Autodesk Inventor part; units mm, degrees
(part 2 of 2)
  spline S15 degree 2 poles (-9.398, 4.6838) (-9.0358, 4.6838) (-8.2948, 4.8649) (-7.9572, 5.0049) knots 0 0 0 1 2 2 2
  spline S16 degree 2 poles (-7.9572, 5.0049) (-7.669, 5.1202) (-7.1338, 5.4495) (-6.9692, 5.5648) knots 0 0 0 1 2 2 2
  line L105 (-6.9692, 5.5648) -> (-6.8951, 5.5648)
  line L106 (-6.8951, 5.5648) -> (-6.8951, 4.1157)
  spline S17 degree 2 poles (-6.8951, 4.1157) (-7.315, 3.9099) (-8.8217, 3.5064) (-9.4968, 3.5064) knots 0 0 0 1 2 2 2
  spline S18 degree 2 poles (-9.4968, 3.5064) (-10.9212, 3.5064) (-12.5267, 5.0131) (-12.5267, 6.2975) knots 0 0 0 1 2 2 2
  spline S19 degree 2 poles (-12.5267, 6.2975) (-12.5267, 6.8986) (-12.2468, 7.9031) (-11.9998, 8.3312) knots 0 0 0 1 2 2 2
  spline S20 degree 2 poles (-11.9998, 8.3312) (-11.7528, 8.7758) (-11.0365, 9.6485) (-10.6413, 10.0684) knots 0 0 0 1 2 2 2
  spline S21 degree 2 poles (-10.6413, 10.0684) (-9.9991, 10.7683) (-8.4265, 12.2668) (-7.9572, 12.7031) knots 0 0 0 1 2 2 2
  line L107 (-7.9572, 12.7031) -> (-12.9466, 12.7031)
  line L108 (-12.9466, 12.7031) -> (-12.9466, 13.8805)
  line L109 (-50.5534, 75.3641) -> (-56.819, 75.3641)
  line L110 (-56.819, 75.3641) -> (-56.819, 76.8049)
  spline S22 degree 2 poles (-56.819, 76.8049) (-56.1439, 77.4389) (-54.9418, 78.6163) (-54.3654, 79.2502) knots 0 0 0 1 2 2 2
  spline S23 degree 2 poles (-54.3654, 79.2502) (-53.2045, 80.5264) (-52.3565, 82.0578) (-52.3565, 82.8729) knots 0 0 0 1 2 2 2
  spline S24 degree 2 poles (-52.3565, 82.8729) (-52.3565, 83.3011) (-52.62, 83.9433) (-52.8587, 84.1491) knots 0 0 0 1 2 2 2
  spline S25 degree 2 poles (-52.8587, 84.1491) (-53.0975, 84.3549) (-53.7232, 84.5608) (-54.102, 84.5608) knots 0 0 0 1 2 2 2
  spline S26 degree 2 poles (-54.102, 84.5608) (-54.4642, 84.5608) (-55.2052, 84.3796) (-55.5428, 84.2397) knots 0 0 0 1 2 2 2
  spline S27 degree 2 poles (-55.5428, 84.2397) (-55.831, 84.1244) (-56.3662, 83.7951) (-56.5308, 83.6798) knots 0 0 0 1 2 2 2
  line L111 (-56.5308, 83.6798) -> (-56.6049, 83.6798)
  line L112 (-56.6049, 83.6798) -> (-56.6049, 85.1289)
  spline S28 degree 2 poles (-56.6049, 85.1289) (-56.185, 85.3347) (-54.6783, 85.7381) (-54.0032, 85.7381) knots 0 0 0 1 2 2 2
  spline S29 degree 2 poles (-54.0032, 85.7381) (-52.5788, 85.7381) (-50.9733, 84.2314) (-50.9733, 82.947) knots 0 0 0 1 2 2 2
  spline S30 degree 2 poles (-50.9733, 82.947) (-50.9733, 82.346) (-51.2532, 81.3415) (-51.5002, 80.9134) knots 0 0 0 1 2 2 2
  spline S31 degree 2 poles (-51.5002, 80.9134) (-51.7472, 80.4688) (-52.4635, 79.596) (-52.8587, 79.1761) knots 0 0 0 1 2 2 2
  spline S32 degree 2 poles (-52.8587, 79.1761) (-53.5009, 78.4763) (-55.0735, 76.9778) (-55.5428, 76.5415) knots 0 0 0 1 2 2 2
  line L113 (-55.5428, 76.5415) -> (-50.5534, 76.5415)
  line L114 (-50.5534, 76.5415) -> (-50.5534, 75.3641)
  line L115 (-12.9466, 13.8805) -> (-6.681, 13.8805)
  line L116 (-6.681, 13.8805) -> (-6.681, 12.4397)
  spline S33 degree 2 poles (-6.681, 12.4397) (-7.3561, 11.8057) (-8.5582, 10.6283) (-9.1346, 9.9943) knots 0 0 0 1 2 2 2
  spline S34 degree 2 poles (-9.1346, 9.9943) (-10.2955, 8.7182) (-11.1435, 7.1868) (-11.1435, 6.3716) knots 0 0 0 1 2 2 2
  spline S35 degree 2 poles (-11.1435, 6.3716) (-11.1435, 5.9435) (-10.88, 5.3013) (-10.6413, 5.0955) knots 0 0 0 1 2 2 2
  spline S36 degree 2 poles (-10.6413, 5.0955) (-10.4025, 4.8896) (-9.7768, 4.6838) (-9.398, 4.6838) knots 0 0 0 1 2 2 2
  spline S37 degree 2 poles (-9.398, 4.6838) (-9.0358, 4.6838) (-8.2948, 4.8649) (-7.9572, 5.0049) knots 0 0 0 1 2 2 2
  spline S38 degree 2 poles (-7.9572, 5.0049) (-7.669, 5.1202) (-7.1338, 5.4495) (-6.9692, 5.5648) knots 0 0 0 1 2 2 2
  line L117 (-6.9692, 5.5648) -> (-6.8951, 5.5648)
  line L118 (-6.8951, 5.5648) -> (-6.8951, 4.1157)
  spline S39 degree 2 poles (-6.8951, 4.1157) (-7.315, 3.9099) (-8.8217, 3.5064) (-9.4968, 3.5064) knots 0 0 0 1 2 2 2
  spline S40 degree 2 poles (-9.4968, 3.5064) (-10.9212, 3.5064) (-12.5267, 5.0131) (-12.5267, 6.2975) knots 0 0 0 1 2 2 2
  spline S41 degree 2 poles (-12.5267, 6.2975) (-12.5267, 6.8986) (-12.2468, 7.9031) (-11.9998, 8.3312) knots 0 0 0 1 2 2 2
  spline S42 degree 2 poles (-11.9998, 8.3312) (-11.7528, 8.7758) (-11.0365, 9.6485) (-10.6413, 10.0684) knots 0 0 0 1 2 2 2
  spline S43 degree 2 poles (-10.6413, 10.0684) (-9.9991, 10.7683) (-8.4265, 12.2668) (-7.9572, 12.7031) knots 0 0 0 1 2 2 2
  line L119 (-7.9572, 12.7031) -> (-12.9466, 12.7031)
  line L120 (-12.9466, 12.7031) -> (-12.9466, 13.8805)
  point P0 (-31.75, 68.8958)
  point P1 (-31.75, 20.0009)
  point P2 (-53.7479, 68.8958)
  point P3 (-9.7521, 20.0042)
  point P4 (-13.4723, 102.9238)
  point P5 (-31.75, 68.8958)
  point P6 (-31.75, 20.0009)
  point P7 (-53.7479, 68.8958)
  point P8 (-9.7521, 20.0042)
  dimension "d103" = 8.4153
  dimension "d105" = 0.508
  dimension "d106" = 0.508
  constraints: 220 point on circle, 170 end point, 120 centre point, 20 perpendicular, 20 tangent, 8 vertical, 4 horizontal, 2 midpoint, 1 parallel, 4 other
  measures "d103" distance of L12.end L14.start
  measures "d105" distance between parallel lines of L15 L7
  measures "d106" distance between parallel lines of L16 L11
extrude "Extrusion20" add sketch "Sketch17" along normal blind 0.4 contours L40 A34 A33 A32 L39 L38 L37 L36 A31 A30 A29 A28 A27 L35 A26 L34 A25 A24 L33 | L56 A58 A57 A56 L55 L54 L53 L52 A55 A54 A53 A52 A51 L51 A50 L50 A49 A48 L49 | L72 A82 A81 A80 L71 L70 L69 L68 A79 A78 A77 A76 A75 L67 A74 L66 A73 A72 L65 | L92 A113 A112 L95 L96 A116 A117 A115 L93 L89 L91 L94 A111 A110 A108 A114 A109 L90 A107 | L97 L98 S0 S1 S2 S3 S4 S5 L99 L100 S6 S7 S8 S9 S10 L101 L102 | L103 L104 S11 S12 S13 S14 S15 S16 L105 L106 S17 S18 S19 S20 S21 L107 L108 bodies 1
sketch "Sketch18" plane through (0, 0, -0.2) normal (0, 0, -1) x (-1, 0, 0)
  line L0 (0, 0) -> (-63.5, 0)
  line L1 (-63.5, 0) -> (-63.5, 88.9)
  line L2 (-63.5, 88.9) -> (0, 88.9)
  line L3 (0, 88.9) -> (0, 0)
  constraints: 8 end point, 2 parallel, 1 horizontal, 1 perpendicular
extrude "Extrusion21" add sketch "Sketch18" along normal blind 0.4 bodies 3
fillet "Fillet2" radius 3.175 8 edges at (63.5, 0, 0.2) (63.5, 88.9, 0.2) (0, 0, 0.2) (0, 88.9, 0.2) (63.5, 0, -0.3) (63.5, 88.9, -0.3) (0, 0, -0.3) (0, 88.9, -0.3)
extrude "Extrusion22" cut sketch "Sketch17" along normal blind 0.4 contours L40 A34 A33 A32 L39 L38 L37 L36 A31 A30 A29 A28 A27 L35 A26 L34 A25 A24 L33 | L44 A41 A40 L47 L48 A44 A45 A43 L45 L41 L43 L46 A39 A38 A36 A42 A37 L42 A35 | L56 A58 A57 A56 L55 L54 L53 L52 A55 A54 A53 A52 A51 L51 A50 L50 A49 A48 L49 | L60 A65 A64 L63 L64 A68 A69 A67 L61 L57 L59 L62 A63 A62 A60 A66 A61 L58 A59 | L72 A82 A81 A80 L71 L70 L69 L68 A79 A78 A77 A76 A75 L67 A74 L66 A73 A72 L65 | L76 A89 A88 L79 L80 A92 A93 A91 L77 L73 L75 L78 A87 A86 A84 A90 A85 L74 A83 | L88 A106 A105 A104 L87 L86 L85 L84 A103 A102 A101 A100 A99 L83 A98 L82 A97 A96 L81 | L92 A113 A112 L95 L96 A116 A117 A115 L93 L89 L91 L94 A111 A110 A108 A114 A109 L90 A107 | L97 L98 S0 S1 S2 S3 S4 S5 L99 L100 S6 S7 S8 S9 S10 L101 L102 | L103 L104 S11 S12 S13 S14 S15 S16 L105 L106 S17 S18 S19 S20 S21 L107 L108 bodies 3
extrude "Extrusion23" add sketch "Sketch17" along normal blind 0.4 contours L44 A41 A40 L47 L48 A44 A45 A43 L45 L41 L43 L46 A39 A38 A36 A42 A37 L42 A35 | L60 A65 A64 L63 L64 A68 A69 A67 L61 L57 L59 L62 A63 A62 A60 A66 A61 L58 A59 | L76 A89 A88 L79 L80 A92 A93 A91 L77 L73 L75 L78 A87 A86 A84 A90 A85 L74 A83 | L88 A106 A105 A104 L87 L86 L85 L84 A103 A102 A101 A100 A99 L83 A98 L82 A97 A96 L81 bodies 4
